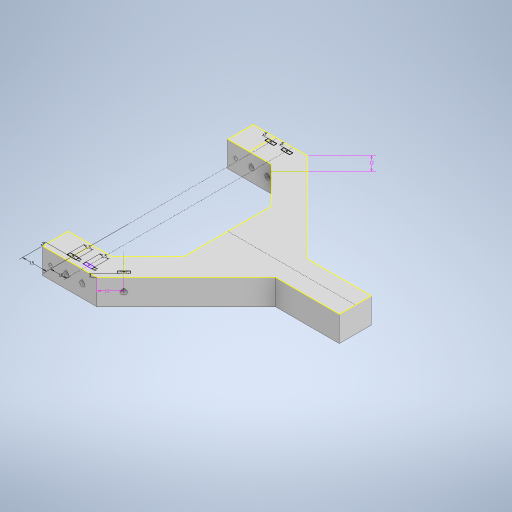
# Autodesk Inventor part: middle_Y
Saved by Autodesk Inventor 2023 (Build 270158000, 158)
## iProperties
Created: 2023-11-20
Part Number: middle_Y
Material: Všeobecné
Document SubType Name: Modeling
Designer: zavrel
Density: 1 g/cm^3
Appearance: Výchozí
Author: zavrel
Autodesk Inventor part; units mm, degrees
ref_plane "YZ Plane" through (0, 0, 0) normal (1, 0, 0) x (0, 1, 0)
ref_plane "XZ Plane" through (0, 0, 0) normal (0, 1, 0) x (-1, 0, 0)
ref_plane "XY Plane" through (0, 0, 0) normal (0, 0, 1) x (1, 0, 0)
sketch "Náčrt1" plane through (0, 0, 0) normal (0, 1, 0) x (-1, 0, 0)
  line L0 (0, 0) -> (0, 10)
  line L1 (0, 10) -> (40, 10)
  line L2 (40, 10) -> (96, 66)
  line L3 (96, 66) -> (130, 66)
  line L4 (130, 66) -> (130, 50)
  line L5 (130, 50) -> (102.6274, 50)
  line L6 (102.6274, 50) -> (80, 27.3726)
  line L7 (80, 27.3726) -> (80, 0)
  line L8 (0, 0) -> (258.3801, 0) construction
  line L9 (0, 0) -> (0, -10)
  line L10 (0, -10) -> (40, -10)
  line L11 (40, -10) -> (96, -66)
  line L12 (96, -66) -> (130, -66)
  line L13 (130, -66) -> (130, -50)
  line L14 (130, -50) -> (102.6274, -50)
  line L15 (102.6274, -50) -> (80, -27.3726)
  line L16 (80, -27.3726) -> (80, 0)
  dimension "d0" = 16
  dimension "d2" = 16
  dimension "d3" = 45
  dimension "d4" = 10
  dimension "d5" = 40
  dimension "d7" = 100
  dimension "d9" = 80
  dimension "d10" = 50
  constraints: 34 end point, 7 symmetric about line, 3 perpendicular, 2 horizontal, 2 parallel, 1 point on line, 1 vertical
  measures "d0" distance of L3.end L4.end
  measures "d2" distance between parallel lines of L6 L2
  measures "d3" angle of L8 L2
  measures "d4" distance between parallel lines of L8 L1
  measures "d5" distance of L9.end L10.end
  measures "d7" distance between parallel lines of L14 L5
  measures "d9" distance between parallel lines of L9 L16
  measures "d10" distance between parallel lines of L16 L13
extrude "Vysunutí1" add sketch "Náčrt1" along normal blind 16
sketch "Náčrt2" plane through (-96, 0, -66) normal (0, 0, -1) x (-1, 0, 0)
  line L0 (0, 0) -> (34, 0) projected
  line L1 (34, 0) -> (34, 16) projected
  line L2 (0, 16) -> (34, 16) projected
  line L3 (0, 0) -> (0, 16) projected
  line L4 (34, 8) -> (0, 8) construction
  circle A0 centre (29, 8) radius 1
  circle A1 centre (19, 8) radius 1.6
  circle A2 centre (9, 8) radius 1.6
  line L5 (19, 8) -> (19, 11.8271) construction
  line L6 (19, 10.2627) -> (20.1314, 9.1314)
  line L7 (19, 10.2627) -> (17.8686, 9.1314)
  line L8 (9, 10.2627) -> (10.1314, 9.1314)
  line L9 (9, 10.2627) -> (7.8686, 9.1314)
  point P0 (-96, 0)
  point P1 (7.8686, 9.1314)
  point P2 (10.1314, 9.1314)
  dimension "d13" = 2
  dimension "d14" = 3.2
  dimension "d15" = 5
  dimension "d16" = 10
  dimension "d17" = 10
  dimension "d22" = 90
  dimension "d23" = 90
  constraints: 12 end point, 4 point on line, 3 centre point, 2 midpoint, 2 point on circle, 2 tangent, 1 equal radius, 1 vertical
  measures "d13" diameter of A0
  measures "d14" diameter of A1
  measures "d15" distance from line of L1 A0.centre
  measures "d16" distance of A0.centre L5.start
  measures "d17" distance of L5.start A2.centre
  measures "d22" angle of L7 L6
  measures "d23" angle of L9 L8
extrude "Vysunutí2" cut sketch "Náčrt2" against normal up to surface (132 mm away) contours A0 | A1 | A1 L7 L6 | A2 | A2 L9 L8
sketch "Náčrt3" plane through (-96, 0, -66) normal (0.7071068, 0, -0.7071068) x (-0.7071068, 0, -0.7071068)
  line L0 (-79.196, 0) -> (0, 0) projected
  line L1 (0, 0) -> (0, 16) projected
  line L2 (-79.196, 16) -> (0, 16) projected
  line L3 (-79.196, 0) -> (-79.196, 16) projected
  line L4 (0, 8) -> (-20.1825, 8) construction
  circle A0 centre (-12, 8) radius 1.6
  line L5 (-12, 8) -> (-12, 19.2417) construction
  line L6 (-12, 10.2627) -> (-10.8686, 9.1314)
  line L7 (-12, 10.2627) -> (-13.1314, 9.1314)
  point P0 (-114.5513, 0)
  dimension "d20" = 3.2
  dimension "d21" = 90
  dimension "d26" = 12
  constraints: 8 end point, 2 point on circle, 2 point on line, 2 tangent, 1 centre point, 1 horizontal, 1 midpoint, 1 vertical
  measures "d20" diameter of A0
  measures "d21" angle of L7 L6
  measures "d26" distance from line of L1 L5.start
extrude "Vysunutí3" cut sketch "Náčrt3" against normal up to surface (16 mm away) contours A0 | A0 L7 L6
sketch "Náčrt4" plane through (-40, 0, 10) normal (0.7071068, 0, 0.7071068) x (0.7071068, 0, -0.7071068)
  line L0 (-79.196, 0) -> (0, 0) projected
  line L1 (0, 0) -> (0, 16) projected
  line L2 (-79.196, 16) -> (0, 16) projected
  line L3 (-79.196, 0) -> (-79.196, 16) projected
  line L4 (-79.196, 8) -> (0, 8) construction
  circle A0 centre (-67.196, 8) radius 1.6
  line L5 (-67.196, 8) -> (-67.196, 16) construction
  line L6 (-67.196, 10.2627) -> (-68.3273, 9.1314)
  line L7 (-67.196, 10.2627) -> (-66.0646, 9.1314)
  point P0 (35.3553, 0)
  dimension "d27" = 3.2
  dimension "d28" = 12
  dimension "d29" = 90
  constraints: 8 end point, 3 point on line, 2 midpoint, 2 point on circle, 2 tangent, 1 centre point, 1 perpendicular
  measures "d27" diameter of A0
  measures "d28" distance from line of L3 L5.start
  measures "d29" angle of L7 L6
extrude "Vysunutí4" cut sketch "Náčrt4" against normal up to surface (16 mm away) contours A0 | A0 L6 L7
sketch "Náčrt5" plane through (0, 16, 0) normal (0, 1, 0) x (1, 0, 0)
  line L0 (-40, 10) -> (-96, 66) projected
  line L1 (-96, 66) -> (-130, 66) projected
  line L2 (-130, 66) -> (-130, 50) projected
  line L3 (-130, 50) -> (-102.6274, 50) projected
  line L4 (-102.6274, 50) -> (-80, 27.3726) projected
  line L5 (-80, 27.3726) -> (-80, -27.3726) projected
  line L6 (-80, -27.3726) -> (-102.6274, -50) projected
  line L7 (-102.6274, -50) -> (-130, -50) projected
  line L8 (-130, -50) -> (-130, -66) projected
  line L9 (-130, -66) -> (-96, -66) projected
  line L10 (-96, -66) -> (-40, -10) projected
  line L11 (-40, -10) -> (0, -10) projected
  line L12 (0, -10) -> (0, 10) projected
  line L13 (0, 10) -> (-40, 10) projected
  line L14 (-115, 66) -> (-115, -77.3891) construction
  line L15 (-105, 66) -> (-105, -72.5981) construction
  line L16 (-102.311, -42.7184) -> (-87.5147, -57.5147) construction
  line L17 (-112.25, -61) -> (-117.75, -61)
  line L18 (-117.75, -61) -> (-117.75, -63)
  line L19 (-117.75, -63) -> (-112.25, -63)
  line L20 (-112.25, -63) -> (-112.25, -61)
  line L21 (-115, -50) -> (-115, -66) projected
  line L22 (-112.25, -61) -> (-117.75, -63) construction
  line L23 (-117.75, -61) -> (-112.25, -63) construction
  line L24 (-102.25, -61) -> (-107.75, -61)
  line L25 (-107.75, -61) -> (-107.75, -63)
  line L26 (-107.75, -63) -> (-102.25, -63)
  line L27 (-102.25, -63) -> (-102.25, -61)
  line L28 (-102.25, -61) -> (-107.75, -63) construction
  line L29 (-107.75, -61) -> (-102.25, -63) construction
  line L30 (-89.1057, -52.0346) -> (-92.9948, -55.9237)
  line L31 (-92.9948, -55.9237) -> (-91.5806, -57.3379)
  line L32 (-91.5806, -57.3379) -> (-87.6915, -53.4489)
  line L33 (-87.6915, -53.4489) -> (-89.1057, -52.0346)
  line L34 (-87.5147, -57.5147) -> (-98.8284, -46.201) projected
  line L35 (-89.1057, -52.0346) -> (-91.5806, -57.3379) construction
  line L36 (-92.9948, -55.9237) -> (-87.6915, -53.4489) construction
  line L37 (-80, 0) -> (0, 0) construction
  line L38 (-87.5147, 57.5147) -> (-98.8284, 46.201) construction
  line L39 (-112.25, 63) -> (-117.75, 63)
  line L40 (-117.75, 63) -> (-117.75, 61)
  line L41 (-117.75, 61) -> (-112.25, 61)
  line L42 (-112.25, 61) -> (-112.25, 63)
  line L43 (-112.25, 63) -> (-117.75, 61) construction
  line L44 (-117.75, 63) -> (-112.25, 61) construction
  line L45 (-116.6, 66) -> (-116.6, 50) projected
  line L46 (-102.25, 63) -> (-107.75, 63)
  line L47 (-107.75, 63) -> (-107.75, 61)
  line L48 (-107.75, 61) -> (-102.25, 61)
  line L49 (-102.25, 61) -> (-102.25, 63)
  line L50 (-102.25, 63) -> (-107.75, 61) construction
  line L51 (-107.75, 63) -> (-102.25, 61) construction
  line L52 (-87.5147, 57.5147) -> (-98.8284, 46.201) projected
  point P0 (-115, -62)
  point P1 (-105, -62)
  point P2 (-90.3431, -54.6863)
  point P3 (-115, 62)
  point P4 (-105, 62)
  point P5 (-105, 62)
  dimension "d32" = 15
  dimension "d33" = 10
  dimension "d34" = 12
  dimension "d35" = 5.5
  dimension "d36" = 2
  dimension "d38" = 3
  dimension "d39" = 5.5
  dimension "d40" = 2
  dimension "d42" = 3
  dimension "d43" = 12
  dimension "d44" = 3
  dimension "d45" = 3
  constraints: 70 end point, 12 midpoint, 10 parallel, 10 point on line, 9 perpendicular, 6 equal length, 3 horizontal, 2 vertical
  measures "d32" distance between parallel lines of L8 L14
  measures "d33" distance between parallel lines of L15 L14
  measures "d34" distance from line of L9.end L16
  measures "d35" distance between parallel lines of L18 L20
  measures "d36" distance of L19.end L17.start
  measures "d38" distance between parallel lines of L9 L19
  measures "d39" distance between parallel lines of L25 L27
  measures "d40" distance of L27.start L27.end
  measures "d42" distance between parallel lines of L10 L32
  measures "d43" distance from line of L0.end L38
  measures "d44" distance between parallel lines of L1 L39
  measures "d45" distance between parallel lines of L1 L46
